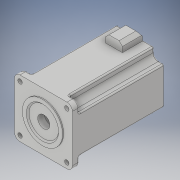
# Autodesk Inventor part: Body
Saved by Autodesk Inventor 2018 (Build 220112000, 112)
## iProperties
Created: 2017-05-16
Part Number: Body
Material: Generic
Document SubType Name: Modeling
Designer: M220404
Density: 1 g/cm^3
Appearance: Default
Author: M220404
Autodesk Inventor part; units mm, degrees
ref_plane "YZ Plane" through (0, 0, 0) normal (1, 0, 0) x (0, 1, 0)
ref_plane "XZ Plane" through (0, 0, 0) normal (0, 1, 0) x (-1, 0, 0)
sketch "Sketch1" plane through (0, 0, 0) normal (0, 0, 1) x (1, 0, 0)
  line L0 (-43, -43) -> (43, -43)
  line L1 (43, -43) -> (43, 43)
  line L2 (43, 43) -> (-43, 43)
  line L3 (-43, 43) -> (-43, -43)
  point P0 (0, 0)
  point P1 (-43, 0)
  point P2 (0, 43)
  dimension "d0" = 86
  dimension "d1" = 86
  constraints: 8 end point, 2 midpoint, 2 parallel, 1 horizontal alignment, 1 perpendicular, 1 vertical, 1 vertical alignment
  measures "d0" distance of L2.end L1.end
  measures "d1" distance of L1.end L0.end
extrude "Extrusion1" add sketch "Sketch1" against normal blind 140
sketch "Sketch2" plane through (0, 0, 0) normal (0, 0, 1) x (1, 0, 0)
  line L0 (-43, 43) -> (43, 43) construction
  line L1 (0, 43) -> (0, -43) construction
  line L2 (43, -43) -> (0, -43) construction
  line L3 (43, 43) -> (43, -43) construction
  line L4 (43, 0) -> (-43, 0) construction
  line L5 (-43, 0) -> (-43, 43) construction
  circle A0 centre (0, 0) radius 30
  point P0 (0, 0)
  dimension "d5" = 60
  constraints: 4 end point, 3 midpoint, 1 centre point, 4 other
  measures "d5" diameter of A0
extrude "Extrusion2" add sketch "Sketch2" along normal blind 1.5
sketch "Sketch3" plane through (0, 0, 1.5) normal (0, 0, 1) x (1, 0, 0)
  line L0 (43, 43) -> (-43, 43) construction
  line L1 (0, 43) -> (0, -43) construction
  line L2 (0, -43) -> (43, -43) construction
  line L3 (43, -43) -> (43, 43) construction
  line L4 (43, 0) -> (-43, 0) construction
  line L5 (-43, 43) -> (-43, 0) construction
  circle A0 centre (0, 0) radius 30 projected
  circle A1 centre (0, 0) radius 7
  point P0 (0, 0)
  dimension "d8" = 14
  constraints: 4 end point, 2 midpoint, 1 centre point, 1 coincident, 4 other
  measures "d8" diameter of A1
extrude "Extrusion3" add sketch "Sketch3" along normal blind 40 contours A1
hole "Hole1" at (0, 0, 41.5) direction (0, 0, -1) diameter 3 depth 13
ref_plane "Work Plane1" through (-7, 0, 1.5) normal (1, 0, 0) x (0, 1, 0)
sketch "Sketch5" plane through (-7, 0, 1.5) normal (1, 0, 0) x (0, 1, 0)
  line L0 (7, 40) -> (-7, 40) projected
  line L1 (-7, 0) -> (7, 0) projected
  line L2 (7, 0) -> (7, 40) projected
  line L3 (-7, 0) -> (-7, 40) projected
  line L4 (7, 40) -> (-7, 40) projected
  line L5 (-2.5, 17.5) -> (-2.5, 40)
  line L6 (-2.5, 40) -> (2.5, 40)
  line L7 (2.5, 40) -> (2.5, 17.5)
  line L8 (30, 0) -> (-30, 0) construction
  arc A0 (-2.5, 17.5) -> (2.5, 17.5) centre (0, 17.5) ccw
  point P0 (0, -1.5)
  point P1 (0, 15)
  constraints: 6 end point, 3 point on circle, 1 centre point, 1 parallel, 1 point on line, 1 tangent
extrude "Extrusion4" cut sketch "Sketch5" along normal blind 2.438 contours L7 A0 L5 L0
sketch "Sketch6" plane through (0, 0, -140) normal (0, 0, -1) x (-1, 0, 0)
  circle A0 centre (0, 0) radius 30 projected
  line L0 (-43, 43) -> (-28, 43)
  line L1 (-28, 43) -> (-28, 35.5)
  line L2 (-35.5, 28) -> (-43, 28)
  line L3 (-43, 28) -> (-43, 43)
  arc A1 (-35.5, 28) -> (-28, 35.5) centre (-35.5, 35.5) ccw
  line L4 (-43, -43) -> (-43, -28)
  line L5 (-43, -28) -> (-35.5, -28)
  line L6 (-28, -35.5) -> (-28, -43)
  line L7 (-28, -43) -> (-43, -43)
  arc A2 (-28, -35.5) -> (-35.5, -28) centre (-35.5, -35.5) ccw
  line L8 (43, -43) -> (28, -43)
  line L9 (28, -43) -> (28, -35.5)
  line L10 (35.5, -28) -> (43, -28)
  line L11 (43, -28) -> (43, -43)
  arc A3 (35.5, -28) -> (28, -35.5) centre (35.5, -35.5) ccw
  line L12 (43, 43) -> (43, 28)
  line L13 (43, 28) -> (35.5, 28)
  line L14 (28, 35.5) -> (28, 43)
  line L15 (28, 43) -> (43, 43)
  arc A4 (28, 35.5) -> (35.5, 28) centre (35.5, 35.5) ccw
  dimension "d71" = 15
  dimension "d72" = 15
  dimension "d75" = 360
  constraints: 32 end point, 8 point on circle, 4 centre point, 2 parallel, 1 horizontal, 1 perpendicular, 45 other
  measures "d71" distance of L2.end L0.start
  measures "d72" distance of L0.start L0.end
sketch "Sketch7" plane through (0, 0, 0) normal (0, 0, 1) x (1, 0, 0)
  circle A0 centre (-34.8, -34.8) radius 3.25
  arc A1 (-6.5383, -2.5) -> (-6.5383, 2.5) centre (0, 0) ccw projected
  circle A2 centre (0, 0) radius 1.5 projected
  circle A3 centre (0, 0) radius 30 projected
  circle A4 centre (0, 0) radius 7 projected
  circle A5 centre (0, 0) radius 30 projected
  line L0 (43, 43) -> (-43, 43) construction
  line L1 (0, 43) -> (0, -43) construction
  line L2 (0, -43) -> (43, -43) construction
  line L3 (-43, 43) -> (-43, 0) construction
  line L4 (-43, 0) -> (43, 0) construction
  line L5 (43, -43) -> (43, 43) construction
  circle A6 centre (-34.8, 34.8) radius 3.25
  circle A7 centre (34.8, -34.8) radius 3.25
  circle A8 centre (34.8, 34.8) radius 3.25
  point P0 (0, 0)
  dimension "d36" = 6.5
  dimension "d37" = 69.6
  dimension "d38" = 69.6
  constraints: 4 centre point, 4 end point, 3 symmetric about line, 2 midpoint, 7 other
  measures "d36" diameter of A0
  measures "d37" distance of A0.centre A6.centre
  measures "d38" distance of A8.centre A6.centre
extrude "Extrusion6" cut sketch "Sketch7" against normal through all contours A0 | A6 | A7 | A8
sketch "Sketch8" plane through (-43, 43, 0) normal (0, 1, 0) x (1, 0, 0)
  line L0 (30.5, 135) -> (55.5, 135)
  line L1 (55.5, 135) -> (55.5, 105)
  line L2 (55.5, 105) -> (30.5, 105)
  line L3 (30.5, 105) -> (30.5, 135)
  line L4 (0, 140) -> (86, 140) projected
  line L5 (43, 135) -> (43, 105) construction
  point P0 (43, 0)
  point P1 (61, 140)
  dimension "d41" = 25
  dimension "d42" = 30
  dimension "d43" = 5
  constraints: 10 end point, 2 midpoint, 2 parallel, 1 horizontal, 1 perpendicular
  measures "d41" distance of L1.end L2.end
  measures "d42" distance of L0.end L1.end
  measures "d43" distance between parallel lines of L4 L0
extrude "Extrusion7" add sketch "Sketch8" along normal blind 13
chamfer "Chamfer1" distance 5 distance2 7 1 edges at (0, 56, -135) measured on face at (-4.1667, 56, -125)
fillet "Fillet1" radius 8 4 edges at (-43, 43, -70) (43, 43, -70) (-43, -43, -70) (43, -43, -70)
chamfer "Chamfer2" distance 5 angle 45 2 edges at (-12.5, 56, -117.5) (12.5, 56, -117.5)
chamfer "Chamfer3" distance 1 angle 45 2 edges at (1.2711, -6.8836, 41.5) (1.2711, 6.8836, 41.5)
sketch "Sketch9" plane through (0, 0, -140) normal (0, 0, -1) x (-1, 0, 0)
  line L0 (43, -35) -> (43, 35) projected
  line L1 (35, 43) -> (-35, 43) projected
  line L2 (-43, 35) -> (-43, -35) projected
  line L3 (-35, -43) -> (35, -43) projected
  arc A0 (-43, -35) -> (-35, -43) centre (-35, -35) ccw projected
  arc A1 (35, -43) -> (43, -35) centre (35, -35) ccw projected
  arc A2 (43, 35) -> (35, 43) centre (35, 35) ccw projected
  arc A3 (-35, 43) -> (-43, 35) centre (-35, 35) ccw projected
  point P0 (0, 0)
extrude "Extrusion8" cut sketch "Sketch9" against normal blind 3
sketch "Sketch10" plane through (0, 0, -137) normal (0, 0, -1) x (-1, 0, 0)
  circle A0 centre (0, 0) radius 1.5 projected
  circle A1 centre (0, 0) radius 28
  point P0 (0, 0)
  dimension "d61" = 56
  constraints: 1 centre point, 1 coincident
  measures "d61" diameter of A1
extrude "Extrusion9" add sketch "Sketch10" along normal blind 3
chamfer "Chamfer4" distance 3 angle 45 1 edges at (28, 0, -140)
fillet "Fillet3" radius 2 4 edges at (43, 0, -137) (0, 43, -137) (-43, 0, -137) (0, -43, -137)
extrude "Extrusion10" cut sketch "Sketch6" against normal blind 130 contours L0 L1 A1 L2 L3 | L4 L5 A2 L6 L7 | L8 L9 A3 L10 L11 | L12 L13 A4 L14 L15
fillet "Fillet4" radius 2 52 edges at (-28, 42.4144, -136.4144) (-28, 38.2503, -137) (-30.1967, 30.1967, -137) (-38.2502, 28, -137) (-42.4144, 28, -136.4144) (-43, 28, -72.5002) (-28, 43, -72.5002) (-43, 31.5, -10) (-31.5, 43, -10) (-40.6569, 40.6569, -10) (-42.4144, -28, -136.4144) (-38.2502, -28, -137) (-30.1967, -30.1967, -137) (-28, -38.2502, -137) (-28, -42.4144, -136.4144) (-28, -43, -72.5002) (-43, -28, -72.5002) (-31.5, -43, -10) (-43, -31.5, -10) (-40.6569, -40.6569, -10) (-39.25, -28, -10) (-28, -39.25, -10) (-30.1967, -30.1967, -10) (-28, 39.25, -10) (-39.25, 28, -10) (-30.1967, 30.1967, -10) (39.25, 28, -10) (28, 39.25, -10) (30.1967, 30.1967, -10) (31.5, 43, -10) (43, 31.5, -10) (40.6569, 40.6569, -10) (28, 42.4144, -136.4144) (28, 38.2503, -137) (30.1967, 30.1967, -137) (38.2503, 28, -137) (42.4144, 28, -136.4144) (43, 28, -72.5002) (28, 43, -72.5002) (43, -31.5, -10) (31.5, -43, -10) (40.6569, -40.6569, -10) (28, -39.25, -10) (39.25, -28, -10) (30.1967, -30.1967, -10) (42.4144, -28, -136.4144) (38.2503, -28, -137) (30.1967, -30.1967, -137) (28, -38.2502, -137) (28, -42.4144, -136.4144) (28, -43, -72.5002) (43, -28, -72.5002)
sketch "Sketch11" plane through (0, 0, 1.5) normal (0, 0, 1) x (1, 0, 0)
  circle A0 centre (0, 0) radius 30 projected
  circle A1 centre (0, 0) radius 22
  point P0 (0, 0)
  dimension "d81" = 8
  constraints: 1 centre point
  measures "d81" radial gap between concentric circles of A0 A1
extrude "Extrusion11" cut sketch "Sketch11" against normal blind 2 contours A1
chamfer "Chamfer5" distance 2 angle 45 1 edges at (-22, 0, 1.5) measured on face at (27.0428, -2.3932, 1.5)
sketch "Sketch13" plane through (0, 0, -0.5) normal (0, 0, 1) x (1, 0, 0)
  circle A0 centre (0, 0) radius 22 projected
  circle A1 centre (0, 0) radius 9
  circle A2 centre (0, 0) radius 1.5 projected
  circle A3 centre (0, 0) radius 7 projected
  circle A4 centre (0, 0) radius 1.5 projected
  circle A5 centre (0, 0) radius 7
  point P0 (0, 0)
  dimension "d90" = 13
  constraints: 2 centre point, 1 coincident
  measures "d90" radial gap between concentric circles of A0 A1
extrude "Extrusion13" cut sketch "Sketch13" against normal blind 10 contours A1 | A2 | A3
sketch "Sketch14" plane through (0, 0, 41.5) normal (0, 0, 1) x (1, 0, 0)
  circle A0 centre (0, 0) radius 1.5 projected
  circle A1 centre (0, 0) radius 7
  point P0 (0, 0)
  constraints: 1 centre point, 1 coincident
extrude "Extrusion14" cut sketch "Sketch14" against normal up to surface (52 mm away)
sketch "Sketch15" plane through (0, 0, 28.5) normal (0, 0, 1) x (1, 0, 0)
  circle A0 centre (0, 0) radius 1.5 projected
  circle A1 centre (0, 0) radius 1.5
  point P0 (0, 0)
  constraints: 1 centre point, 1 coincident
extrude "Extrusion15" cut sketch "Sketch15" against normal up to surface (39 mm away)
body "Solid1"
